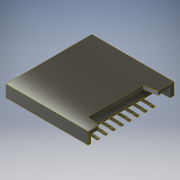
# Autodesk Inventor part: uSDCard
Saved by Autodesk Inventor 2016 (Build 200138000, 138)
## iProperties
Created: 2017-03-03
Part Number: uSDCard
Material: Generic
Document SubType Name: Modeling
Designer: jfixelle
Density: 1 g/cm^3
Appearance: Silver
Author: jfixelle
Autodesk Inventor part; units mm, degrees
ref_plane "YZ Plane" through (0, 0, 0) normal (1, 0, 0) x (0, 1, 0)
ref_plane "XZ Plane" through (0, 0, 0) normal (0, 1, 0) x (-1, 0, 0)
ref_plane "XY Plane" through (0, 0, 0) normal (0, 0, 1) x (1, 0, 0)
sketch "Sketch2" plane through (0, 0, 0) normal (0, 1, 0) x (-1, 0, 0)
  line L0 (11.45, 1.45) -> (0, 1.45)
  line L1 (0, 1.45) -> (0, -10.5)
  line L2 (0, -10.5) -> (11.45, -10.5)
  line L3 (11.45, -10.5) -> (11.45, 1.45)
  line L4 (1.75, 0) -> (1.75, -8.25)
  line L5 (0, 0) -> (1.75, 0) construction
  line L6 (1.75, -8.25) -> (0, -8.25) construction
  line L7 (0, 0) -> (1.75, -0.3086)
  line L8 (0, -8.25) -> (1.75, -7.9414)
  line L9 (0, 0) -> (0, -8.25)
  dimension "d9" = 0
  dimension "d10" = 11.45
  dimension "d11" = 11.95
  dimension "d12" = 10.5
  dimension "d13" = 1.75
  dimension "d14" = 8.25
  dimension "d15" = 10
  dimension "d16" = 10
  constraints: 20 end point, 3 point on line, 2 horizontal, 2 parallel, 2 perpendicular, 1 vertical
  measures "d9" distance from line of L1 L5.start
  measures "d10" distance of L1.end L2.end
  measures "d11" distance of L2.end L0.start
  measures "d12" distance from line of L5.start L2
  measures "d13" distance between parallel lines of L1 L4
  measures "d14" distance between parallel lines of L5 L6
  measures "d15" angle of L6 L8
  measures "d16" angle of L5 L7
extrude "Extrusion2" add sketch "Sketch2" along normal blind 1.68 contours L3 L2 L1 L8 L4 L7 L0
sketch "Sketch3" plane through (0, 0, 1.45) normal (1, 0, 0) x (0, 0, -1)
  line L0 (11.95, 0) -> (0, 0) projected
  line L1 (11.3835, 0) -> (0.3835, 0)
  line L2 (0.3835, 0) -> (0.3835, 1.15)
  line L3 (0.3835, 1.15) -> (11.3835, 1.15)
  line L4 (11.3835, 1.15) -> (11.3835, 0)
  point P0 (1.45, 0)
  dimension "d19" = 11
  dimension "d20" = 1.15
  constraints: 8 end point, 2 parallel, 1 horizontal, 1 perpendicular, 1 point on line
  measures "d19" distance of L2.end L3.end
  measures "d20" distance of L1.end L2.end
extrude "Extrusion3" cut sketch "Sketch3" against normal blind 9.15
sketch "Sketch4" plane through (-1.75, 1.68, -0.3086) normal (1, 0, 0) x (0, 0, -1)
  line L0 (-1.3751, -1.68) -> (-1.3751, -0.53) projected
  line L1 (9.6249, -1.68) -> (-1.3751, -1.68) projected
  line L2 (-1.3751, -1.48) -> (9.6249, -1.48)
  line L3 (9.6249, -1.48) -> (9.6249, -1.68)
  line L4 (9.6249, -1.68) -> (-1.3751, -1.68)
  line L5 (-1.3751, -1.68) -> (-1.3751, -1.48)
  line L6 (0, -0.53) -> (7.6329, -0.53) projected
  line L7 (3.8164, -0.53) -> (5.5042, -0.53)
  point P0 (-0.3086, -1.68)
  dimension "d23" = 0.95
  constraints: 10 end point, 2 parallel, 2 point on line, 1 horizontal, 1 midpoint, 1 perpendicular
  measures "d23" distance between parallel lines of L2 L6
extrude "Extrusion4" add sketch "Sketch4" against normal up to next
sketch "Sketch5" plane through (0, 0, 0) normal (0, 0, 1) x (1, 0, 0)
  line L0 (-2, 0.15) -> (-0.4808, 0.15)
  line L1 (-0.4808, 0.15) -> (-0.4467, 0.1)
  line L2 (-0.4467, 0.1) -> (0, 0.1)
  line L3 (0, 0.1) -> (0, -0.05)
  line L4 (0, -0.05) -> (-0.5, -0.05)
  line L5 (-0.5, -0.05) -> (-0.5341, 0)
  line L6 (-0.5341, 0) -> (-2, 0)
  line L7 (-2, 0) -> (-2, 0.15)
  point P0 (0, 0)
  dimension "d26" = 0
  dimension "d27" = 0.5
  dimension "d28" = 2
  dimension "d29" = 0.05
  dimension "d30" = 0.15
  dimension "d32" = 0.15
  dimension "d33" = 0.2
  constraints: 16 end point, 3 parallel, 3 perpendicular, 1 horizontal
  measures "d26" distance from line of point (0, 0) L3
  measures "d27" distance of L3.end L4.end
  measures "d28" distance between parallel lines of L3 L7
  measures "d29" distance from line of point (0, 0) L4
  measures "d30" distance of L2.end L3.end
  measures "d32" distance between parallel lines of L6 L0
  measures "d33" distance between parallel lines of L4 L0
extrude "Extrusion5" add sketch "Sketch5" along normal mid plane 0.3
pattern_linear "Rectangular Pattern1" count 8 spacing 1.1 along (0, 0, -1) of "Extrusion5"
body "Solid2"
